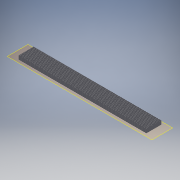
# Autodesk Inventor part: Fin
Saved by Autodesk Inventor 2016 (Build 200138000, 138)
## iProperties
Created: 2017-06-28
Part Number: Fin
Material: Generic
Document SubType Name: Modeling
Designer: Roeder
Density: 1 g/cm^3
Appearance: Default
Author: Roeder
Autodesk Inventor part; units mm, degrees
ref_plane "YZ Plane" through (0, 0, 0) normal (1, 0, 0) x (0, 1, 0)
ref_plane "XZ Plane" through (0, 0, 0) normal (0, 1, 0) x (-1, 0, 0)
ref_plane "XY Plane" through (0, 0, 0) normal (0, 0, 1) x (1, 0, 0)
ref_plane "Work Plane1" through (0, 0, 0) normal (0, 0, 1) x (1, 0, 0)
sketch "Sketch1" plane through (0, 0, 0) normal (0, 0, 1) x (1, 0, 0)
  arc A0 (3437.5, 230) -> (3437.5, 220) centre (3437.5, 225) ccw projected
  line L0 (3437.5, 230) -> (3452.5, 230) projected
  arc A1 (3452.5, 220) -> (3452.5, 230) centre (3452.5, 225) ccw projected
  line L1 (3452.5, 220) -> (3437.5, 220) projected
  arc A2 (2192.5, 230) -> (2192.5, 220) centre (2192.5, 225) ccw projected
  line L2 (2192.5, 230) -> (2207.5, 230) projected
  arc A3 (2207.5, 220) -> (2207.5, 230) centre (2207.5, 225) ccw projected
  line L3 (2207.5, 220) -> (2192.5, 220) projected
  arc A4 (942.5, 230) -> (942.5, 220) centre (942.5, 225) ccw projected
  line L4 (942.5, 230) -> (957.5, 230) projected
  arc A5 (957.5, 220) -> (957.5, 230) centre (957.5, 225) ccw projected
  line L5 (957.5, 220) -> (942.5, 220) projected
  arc A6 (-7.5, 230) -> (-7.5, 220) centre (-7.5, 225) ccw projected
  line L6 (-7.5, 230) -> (7.5, 230) projected
  arc A7 (7.5, 220) -> (7.5, 230) centre (7.5, 225) ccw projected
  line L7 (7.5, 220) -> (-7.5, 220) projected
  arc A8 (-7.5, -220) -> (-7.5, -230) centre (-7.5, -225) ccw projected
  line L8 (-7.5, -220) -> (7.5, -220) projected
  arc A9 (7.5, -230) -> (7.5, -220) centre (7.5, -225) ccw projected
  line L9 (7.5, -230) -> (-7.5, -230) projected
  arc A10 (942.5, -220) -> (942.5, -230) centre (942.5, -225) ccw projected
  line L10 (942.5, -220) -> (957.5, -220) projected
  arc A11 (957.5, -230) -> (957.5, -220) centre (957.5, -225) ccw projected
  line L11 (957.5, -230) -> (942.5, -230) projected
  arc A12 (2192.5, -220) -> (2192.5, -230) centre (2192.5, -225) ccw projected
  line L12 (2192.5, -220) -> (2207.5, -220) projected
  arc A13 (2207.5, -230) -> (2207.5, -220) centre (2207.5, -225) ccw projected
  line L13 (2207.5, -230) -> (2192.5, -230) projected
  arc A14 (3437.5, -220) -> (3437.5, -230) centre (3437.5, -225) ccw projected
  line L14 (3437.5, -220) -> (3452.5, -220) projected
  arc A15 (3452.5, -230) -> (3452.5, -220) centre (3452.5, -225) ccw projected
  line L15 (3452.5, -230) -> (3437.5, -230) projected
  line L16 (22.5, -250) -> (22.5, -200) projected
  line L17 (22.5, -200) -> (927.5, -200) projected
  line L18 (927.5, -200) -> (927.5, -250) projected
  line L19 (927.5, -250) -> (972.5, -250) projected
  line L20 (972.5, -250) -> (972.5, -200) projected
  line L21 (972.5, -200) -> (2177.5, -200) projected
  line L22 (2177.5, -200) -> (2177.5, -250) projected
  line L23 (2177.5, -250) -> (2222.5, -250) projected
  line L24 (2222.5, -250) -> (2222.5, -200) projected
  line L25 (2222.5, -200) -> (3422.5, -200) projected
  line L26 (3422.5, -200) -> (3422.5, -250) projected
  line L27 (3422.5, -250) -> (3467.5, -250) projected
  line L28 (3467.5, -250) -> (3467.5, 250) projected
  line L29 (3467.5, 250) -> (3422.5, 250) projected
  line L30 (3422.5, 250) -> (3422.5, 200) projected
  line L31 (3422.5, 200) -> (2222.5, 200) projected
  line L32 (2222.5, 200) -> (2222.5, 250) projected
  line L33 (2222.5, 250) -> (2177.5, 250) projected
  line L34 (2177.5, 250) -> (2177.5, 200) projected
  line L35 (2177.5, 200) -> (972.5, 200) projected
  line L36 (972.5, 200) -> (972.5, 245) projected
  line L37 (972.5, 245) -> (927.5, 245) projected
  line L38 (927.5, 245) -> (927.5, 200) projected
  line L39 (927.5, 200) -> (22.5, 200) projected
  line L40 (22.5, 200) -> (22.5, 250) projected
  line L41 (22.5, 250) -> (-22.5, 250) projected
  line L42 (-22.5, 250) -> (-22.5, -250) projected
  line L43 (-22.5, -250) -> (22.5, -250) projected
  line L44 (24.5, -200) -> (24.5, 200) projected
  line L45 (24.5, 200) -> (22.5, 200) projected
  line L46 (22.5, 200) -> (22.5, -200) projected
  line L47 (22.5, -200) -> (24.5, -200) projected
  line L48 (971.5, 200) -> (971.5, -200) projected
  line L49 (971.5, -200) -> (973.5, -200) projected
  line L50 (973.5, -200) -> (973.5, 200) projected
  line L51 (973.5, 200) -> (971.5, 200) projected
  line L52 (2221.5, 200) -> (2221.5, -200) projected
  line L53 (2221.5, -200) -> (2223.5, -200) projected
  line L54 (2223.5, -200) -> (2223.5, 200) projected
  line L55 (2223.5, 200) -> (2221.5, 200) projected
  line L56 (3423.5, -200) -> (3423.5, 200) projected
  line L57 (3423.5, 200) -> (3421.5, 200) projected
  line L58 (3421.5, 200) -> (3421.5, -200) projected
  line L59 (3421.5, -200) -> (3423.5, -200) projected
  line L60 (-260.4101, 0) -> (3860.6378, 0) construction
  line L61 (29.5, 200) -> (29.5, -200) construction
  line L62 (29.25, 200) -> (29.75, 200)
  line L63 (29.75, 200) -> (29.75, -200)
  line L64 (29.75, -200) -> (29.25, -200)
  line L65 (29.25, -200) -> (29.25, 200)
  point P0 (0, 0)
  dimension "d2" = 5
  dimension "d3" = 0.5
  constraints: 12 end point, 3 point on line, 2 horizontal, 2 parallel, 2 perpendicular, 1 other
  measures "d2" distance from line of L44 L61.start
  measures "d3" distance of L63.end L64.end
extrude "Extrusion1" add sketch "Sketch1" along normal blind 100 contours L65 L39 L63 L17
pattern_linear "Rectangular Pattern1" count 169 spacing 20 along (1, 0, 0) of "Extrusion1"
body "Solid1"
